Cat Water Bowl anti-tip bracket (Autodesk Fusion 360 design; units mm, degrees)
Autodesk Fusion 360 part; units mm, degrees
sketch "Sketch1" plane through (0, 0, 0) normal (0, 0, 1) x (1, 0, 0)
  line L0 (0, 0) -> (0, 116)
  line L1 (0, 116) -> (45, 116)
  line L2 (45, 116) -> (45, 111)
  line L3 (45, 111) -> (5, 111)
  line L4 (5, 111) -> (5, -5)
  line L5 (5, -5) -> (-30, -5)
  line L6 (-30, -5) -> (-30, 0)
  line L7 (-30, 0) -> (0, 0)
  dimension "d1" = 116
  dimension "d2" = 5
  dimension "d3" = 5
  dimension "d4" = 40
  dimension "d5" = 5
  dimension "d6" = 30
  constraint coincident L0.start L7.end
  constraint vertical L0
  constraint perpendicular L0 L1
  constraint perpendicular L1 L2
  constraint perpendicular L0 L3
  constraint perpendicular L1 L4
  constraint perpendicular L4 L5
  constraint perpendicular L5 L6
  constraint perpendicular L6 L7
  measures "d1" distance of L3 L5
  measures "d2" distance of L1.end L2.end
  measures "d3" distance of L5.end L6.end
  measures "d4" distance of L2.end L3.end
  measures "d5" distance of L0 L4
  measures "d6" distance of L6.end L0.start
extrude "Extrude1" add sketch "Sketch1" along normal blind 13 makes body 1
sketch "Sketch2" plane through (0, 0, 0) normal (0, 1, 0) x (-1, 0, 0)
  line L0 (0, 0) -> (30, 0)
  line L1 (30, 0) -> (30, 13)
  line L2 (30, 13) -> (0, 13)
  line L3 (0, 13) -> (0, 0)
  line L4 (30, 6.5) -> (0, 6.5) construction
  line L5 (15, 6.5) -> (15, 0) construction
  point P0 (8, 6.5)
  point P1 (22, 6.5)
  dimension "d9" = 14
  dimension "d10" = 8
  constraint midpoint L1 L4.start
  constraint midpoint L3 L4.end
  constraint midpoint L4 L5.start
  constraint midpoint L0 L5.end
  constraint coincident L4 P0
  constraint symmetric L5 P0 P1
  measures "d9" distance of P0 P1
  measures "d10" distance of L4.start P1
hole "Hole1" at (-22, 0, 6.5) at (-8, 0, 6.5) direction (0, -1, 0) diameter 4.2 depth 5 tip angle 180 countersink diameter 8 countersink angle 80 bodies 1
fillet "Fillet1" radius 2 7 edges at (-30, 0, 6.5) (0, 0, 6.5) (0, 116, 6.5) (45, 116, 6.5) (5, 111, 6.5) (45, 111, 6.5) (5, -5, 6.5) on bodies 1
sketch "Sketch3" plane through (0, -5, 0) normal (0, -1, 0) x (1, 0, 0)
  line L0 (3, 0) -> (3, 13)
  line L1 (3, 13) -> (-30, 13)
  line L2 (-30, 13) -> (-30, 0)
  line L3 (-30, 0) -> (3, 0)
  circle A0 centre (-8, 6.5) radius 2.1
  circle A1 centre (-22, 6.5) radius 2.1
  circle A2 centre (-22, 6.5) radius 2.1
  circle A3 centre (-8, 6.5) radius 2.1
  line L4 (-22, 6.5) -> (-22, 6.8101)
  line L5 (-22, 6.8101) -> (-22, 9.4698) construction
  line L6 (-22, 9.4698) -> (-20.5151, 7.9849)
  line L7 (-22, 9.4698) -> (-23.4849, 7.9849)
  line L8 (-8, 6.5) -> (-8, 6.7678) construction
  line L9 (-8, 6.7678) -> (-8, 9.4698) construction
  line L10 (-8, 9.4698) -> (-6.5151, 7.9849)
  line L11 (-8, 9.4698) -> (-9.4849, 7.9849)
  constraint coincident A1.centre A2.centre
  constraint vertical L4
  constraint parallel L4 L5
  constraint coincident A1 L6.end
  constraint tangent A1 L6
  constraint symmetric L6.start L5 L7.start
  constraint symmetric L5 L6.end L7.end
  constraint perpendicular L6 L7
  constraint coincident A0.centre A3.centre
  constraint perpendicular L1 L8
  constraint perpendicular L1 L9
  constraint coincident A3 L10.end
  constraint tangent A0 L10
  constraint symmetric L10.start L9 L11.start
  constraint symmetric L9 L10.end L11.end
  constraint perpendicular L10 L11
extrude "Extrude2" cut sketch "Sketch3" against normal blind 5 contours A0 A3 L10 L11 | A1 A2 L6 L7 bodies 1
copy_body "Body->Comp1" bodies 1 removing the originals makes body 2 in component "Cat Water Bowl anti-tip bracket"
sketch "Base Sketch" plane through (0, 0, 0) normal (0, 0, 1) x (1, 0, 0) in component "v2 Anti-tip Bracket"
  line L0 (0, 0) -> (239, 0)
  line L1 (239, 0) -> (239, 115)
  line L2 (239, 115) -> (0, 115)
  line L3 (0, 115) -> (0, 0)
  line L4 (244, -5) -> (244, 120)
  line L5 (244, 120) -> (-5, 120)
  line L6 (-5, 120) -> (-5, -5)
  line L7 (-5, -5) -> (244, -5)
  dimension "d21" = 239
  dimension "d22" = 115
  dimension "d23" = 5
  dimension "d41" = 249
  constraint horizontal L0
  constraint vertical L1
  constraint horizontal L2
  constraint vertical L3
  constraint coincident L0.start L3.end
  measures "d21" distance of L0.start L0.end
  measures "d22" distance of L0.start L2.end
  measures "d41" distance of L4 L6
extrude "Extrude1'" add sketch "Base Sketch" along normal blind 13 separate body makes body 3 in component "v2 Anti-tip Bracket"
sketch "Hole positions and Teardrops" plane through (0, 115, 0) normal (0, -1, 0) x (1, 0, 0) in component "v2 Anti-tip Bracket"
  line L0 (0, 0) -> (239, 0)
  line L1 (239, 0) -> (239, 13)
  line L2 (239, 13) -> (0, 13)
  line L3 (0, 13) -> (0, 0)
  line L4 (-5, 0) -> (244, 0)
  line L5 (244, 0) -> (244, 13)
  line L6 (244, 13) -> (-5, 13)
  line L7 (-5, 13) -> (-5, 0)
  line L8 (119.5, 13) -> (119.5, 32.1039) construction
  circle A0 centre (20.5, 6.5) radius 2
  circle A1 centre (34.5, 6.5) radius 2
  line L9 (-5, 6.5) -> (34.5, 6.5) construction
  circle A2 centre (218.5, 6.5) radius 2
  circle A3 centre (204.5, 6.5) radius 2
  line L10 (218.5, 9.3284) -> (217.0858, 7.9142)
  line L11 (218.5, 6.5) -> (218.5, 9.3284) construction
  line L12 (218.5, 9.3284) -> (219.9142, 7.9142)
  line L13 (219, 8.8284) -> (218, 8.8284)
  line L14 (204.5, 6.5) -> (204.5, 9.3284) construction
  line L15 (204.5, 9.3284) -> (205.9142, 7.9142)
  line L16 (204.5, 9.3284) -> (203.0858, 7.9142)
  line L17 (205, 8.8284) -> (204, 8.8284)
  line L18 (20.5, 9.3284) -> (21.9142, 7.9142)
  line L19 (20, 8.8284) -> (21, 8.8284)
  line L20 (20.5, 9.3284) -> (19.0858, 7.9142)
  line L21 (34.5, 9.3284) -> (33.0858, 7.9142)
  line L22 (34, 8.8284) -> (35, 8.8284)
  line L23 (34.5, 9.3284) -> (35.9142, 7.9142)
  dimension "d26" = 4
  dimension "d27" = 14
  dimension "d28" = 85
  dimension "d36" = 1
  dimension "d38" = 1
  constraint midpoint L6 L8.start
  constraint perpendicular L6 L8
  constraint equal A0 A1
  constraint midpoint L7 L9.start
  constraint coincident A1.centre L9.end
  constraint perpendicular L7 L9
  constraint coincident A0.centre L9
  constraint symmetric L8 A0 A2
  constraint symmetric L8 A1 A3
  constraint coincident A2 L10.end
  constraint tangent A2 L10
  constraint coincident A2.centre L11.start
  constraint perpendicular L6 L11
  constraint coincident A2 L12.end
  constraint tangent A2 L12
  constraint coincident L12 L13.start
  constraint coincident L10 L13.end
  constraint perpendicular L11 L13
  constraint coincident A3.centre L14.start
  constraint vertical L14
  constraint coincident A3 L15.end
  constraint tangent A3 L15
  constraint coincident A3 L16.end
  constraint tangent A3 L16
  constraint coincident L15 L17.start
  constraint coincident L16 L17.end
  constraint perpendicular L14 L17
  constraint perpendicular L15 L16
  constraint perpendicular L10 L12
  constraint symmetric L8 L10.start L18.start
  constraint symmetric L8 L10.end L18.end
  constraint symmetric L8 L12.end L20.end
  constraint symmetric L8 L13.start L19.start
  constraint symmetric L8 L13.end L19.end
  constraint symmetric L8 L14.end L21.start
  constraint symmetric L8 L15.end L21.end
  constraint symmetric L8 L16.end L23.end
  constraint symmetric L8 L17.start L22.start
  constraint symmetric L8 L17.end L22.end
  measures "d26" diameter of A0
  measures "d27" distance of A0.centre A1.centre
  measures "d28" distance of L8 A1.centre
  measures "d36" distance of L13.start L13.end
  measures "d38" distance of L17.start L17.end
hole "Hole1'" at (34.5, 115, 6.5) at (20.5, 115, 6.5) at (218.5, 115, 6.5) at (204.5, 115, 6.5) direction (0, 1, 0) diameter 4 depth 5 tip angle 118 countersink diameter 6 countersink angle 82.5 bodies 3 in component "v2 Anti-tip Bracket"
fillet "Fillet1'" radius 2 6 edges at (0, 115, 6.5) (239, 115, 6.5) (239, 0, 6.5) (0, 0, 6.5) (244, -5, 6.5) (-5, -5, 6.5) on bodies 3 in component "v2 Anti-tip Bracket"
extrude "Extrude2'" cut sketch "Hole positions and Teardrops" against normal blind 5 contours A0 L18 L19 L20 | A1 L21 L22 L23 | A2 L10 L12 L13 | A3 L15 L16 L17 bodies 3 in component "v2 Anti-tip Bracket"
component "Cat Water Bowl anti-tip bracket" placed x (1, 0, 0) y (0, 1, 0) z (0, 0, 1) at (0, 0, 0)
component "v2 Anti-tip Bracket" placed x (1, 0, 0) y (0, 1, 0) z (0, 0, 1) at (0, 0, 0)
equation "d3 = d2"
equation "d5 = d2"
named bodies: "Cat Water Bowl anti-tip bracket", "v2"
